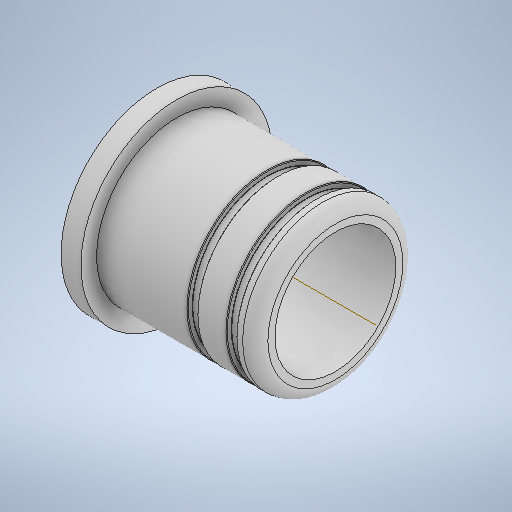
# Autodesk Inventor part: PVCTOP3
Saved by Autodesk Inventor 2025.2 (Build 292293000, 293)
## iProperties
Created: 2025-02-05
Part Number: PVCTOP3
Material: Generic
Document SubType Name: Modeling
Designer: ppita
Density: 1 g/cm^3
Appearance: Default
Author: ppita
Autodesk Inventor part; units mm, degrees
ref_plane "YZ Plane" through (0, 0, 0) normal (1, 0, 0) x (0, 1, 0)
ref_plane "XZ Plane" through (0, 0, 0) normal (0, 1, 0) x (-1, 0, 0)
ref_plane "XY Plane" through (0, 0, 0) normal (0, 0, 1) x (1, 0, 0)
sketch "Sketch1" plane through (0, 0, 0) normal (1, 0, 0) x (0, 1, 0)
  circle A0 centre (0, 0) radius 24.13
  dimension "d0" = 48.26
  constraints: 1 centre point, 1 coincident
  measures "d0" diameter of A0
extrude "Extrusion1" add sketch "Sketch1" along normal blind 5
sketch "Sketch2" plane through (5, 0, 0) normal (1, 0, 0) x (0, 0, -1)
  circle A0 centre (0, 0) radius 20.1803
  dimension "d3" = 40.3606
  constraints: 1 centre point, 1 coincident
  measures "d3" diameter of A0
extrude "Extrusion2" add sketch "Sketch2" along normal blind 40
sketch "Sketch3" plane through (45, 0, 0) normal (1, 0, 0) x (0, 0, -1)
  circle A0 centre (0, 0) radius 15.24
  dimension "d6" = 30.48
  constraints: 1 centre point, 1 coincident
  measures "d6" diameter of A0
extrude "Extrusion3" cut sketch "Sketch3" against normal blind 40
sketch "Sketch4" plane through (0, 0, 0) normal (-1, 0, 0) x (0, 0, 1)
  circle A0 centre (0, 0) radius 8.275
  dimension "d9" = 16.55
  constraints: 1 centre point, 1 coincident
  measures "d9" diameter of A0
extrude "Extrusion4" cut sketch "Sketch4" against normal blind 40
sketch "Sketch5" plane through (0, 0, 0) normal (0, 1, 0) x (-1, 0, 0)
  point P0 (0, 0)
sketch "Sketch6" plane through (0, 0, 0) normal (0, 1, 0) x (-1, 0, 0)
  line L0 (-30.2501, -20.1803) -> (-32.6631, -20.1803)
  line L1 (-5, -20.1803) -> (-45, -20.1803) projected
  line L2 (-32.6631, -20.1803) -> (-32.6631, -18.9611)
  line L3 (-32.6631, -18.9611) -> (-30.2501, -18.9611)
  line L4 (-30.2501, -18.9611) -> (-30.2501, -20.1803)
  line L5 (-32.6631, -18.9611) -> (-32.6631, 0)
  line L6 (-32.6631, 0) -> (-30.2501, 0)
  line L7 (-30.2501, -20.1803) -> (-32.6631, -20.1803)
  line L8 (-5, -20.1803) -> (-45, -20.1803) projected
  line L9 (-5, -20.1803) -> (-45, -20.1803) projected
  line L10 (-37.789, -20.1803) -> (-40.202, -20.1803)
  line L11 (-5, -20.1803) -> (-45, -20.1803) projected
  line L12 (-40.202, -20.1803) -> (-40.202, -18.9611)
  line L13 (-40.202, -18.9611) -> (-37.789, -18.9611)
  line L14 (-37.789, -18.9611) -> (-37.789, -20.1803)
  line L15 (-40.202, -18.9611) -> (-40.202, 0)
  line L16 (-40.202, 0) -> (-37.482, 0)
  line L17 (-40.202, -20.1803) -> (-37.789, -20.1803)
  point P0 (0, 0)
  dimension "d12" = 2.413
  dimension "d13" = 1.2192
  dimension "d14" = 2.413
  dimension "d15" = 2.413
  dimension "d16" = 1.2192
  constraints: 28 end point, 6 perpendicular, 3 vertical, 2 horizontal, 1 collinear, 1 point on line, 5 other
  measures "d12" distance of L0.start L0.end
  measures "d13" distance of L0.end L2.end
  measures "d14" distance of L0.start L0.end
  measures "d15" distance of L10.start L10.end
  measures "d16" distance of L10.end L12.end
revolve "Revolution1" cut sketch "Sketch6" angle 360 about axis through (40.202, 0, 0) along (-1, 0, 0) contours L1 L12 L13 L14
sketch "Sketch7" plane through (0, 0, 0) normal (0, 1, 0) x (-1, 0, 0)
  line L0 (-5, -20.1803) -> (-37.789, -20.1803) projected
  line L1 (-27.9619, -20.1803) -> (-30.3749, -20.1803)
  line L2 (-30.3749, -20.1803) -> (-30.3749, -18.9611)
  line L3 (-30.3749, -18.9611) -> (-27.9619, -18.9611)
  line L4 (-27.9619, -18.9611) -> (-27.9619, -20.1803)
  line L5 (-30.3749, -18.9611) -> (-30.3749, 0)
  line L6 (-30.3749, 0) -> (-27.4344, 0)
  line L7 (7.5578, 0) -> (-45.3468, 0) projected
  point P0 (0, 0)
  dimension "d18" = 2.413
  dimension "d19" = 1.2192
  constraints: 12 end point, 4 perpendicular, 3 point on line
  measures "d18" distance of L1.start L1.end
  measures "d19" distance of L1.end L2.end
revolve "Revolution2" cut sketch "Sketch7" angle 360 about axis through (0, 0, 0) along (1, 0, 0)
fillet "Fillet1" radius 3.175 1 edges at (45, 0, 20.1803)
fillet "Fillet2" radius 0.1778 1 edges at (40.202, 0, 20.1803)
fillet "Fillet3" radius 0.1778 1 edges at (37.789, 0, 20.1803)
fillet "Fillet4" radius 0.1778 1 edges at (30.3749, 0, 20.1803)
fillet "Fillet5" radius 0.1778 1 edges at (27.9619, 0, 20.1803)
fillet "Fillet6" radius 0.0508 1 edges at (30.3749, 0, 18.9611)
fillet "Fillet7" radius 0.0508 1 edges at (27.9619, 0, 18.9611)
fillet "Fillet8" radius 0.0508 1 edges at (37.789, 0, 18.9611)
fillet "Fillet9" radius 0.0508 1 edges at (40.202, 0, 18.9611)
thread "Thread2" size "M16x1.5" class "6H" standard "ISO Metric profile" length 20.1676
body "Solid1"
